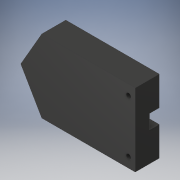
# Autodesk Inventor part: TARM05
Saved by Autodesk Inventor 2017 (Build 210142000, 142)
## iProperties
Created: 2018-10-19
Part Number: TARM05
Material: ABS Plastic
Document SubType Name: Modeling
Designer: Dell
Density: 1.06 g/cm^3
Appearance: Smooth - Black
Author: Dell
Autodesk Inventor part; units mm, degrees
ref_plane "YZ Plane" through (0, 0, 0) normal (1, 0, 0) x (0, 1, 0)
ref_plane "XZ Plane" through (0, 0, 0) normal (0, 1, 0) x (-1, 0, 0)
ref_plane "XY Plane" through (0, 0, 0) normal (0, 0, 1) x (1, 0, 0)
sketch "Sketch1" plane through (0, 0, 0) normal (0, 0, 1) x (1, 0, 0)
  line L0 (-56, 0) -> (-28, 48.4974)
  line L1 (-28, 48.4974) -> (28, 48.4974)
  line L2 (28, 48.4974) -> (56, 0)
  line L3 (56, 0) -> (28, -48.4974)
  line L4 (28, -48.4974) -> (-28, -48.4974)
  line L5 (-28, -48.4974) -> (-56, 0)
  line L6 (28, 48.4974) -> (76, 48.4974)
  line L7 (76, 48.4974) -> (76, -48.4974)
  line L8 (76, -48.4974) -> (28, -48.4974)
  point P0 (0, 0)
  point P1 (0, 0)
  dimension "d0" = 112
  dimension "d1" = 20
  constraints: 18 end point, 2 perpendicular, 1 coincident, 1 horizontal, 1 horizontal alignment, 13 other
  measures "d0" distance of L2.end L0.start
  measures "d1" distance from line of L2.end L7
extrude "Extrusion1" add sketch "Sketch1" along normal blind 5
sketch "Sketch2" plane through (0, 0, 0) normal (0, 0, -1) x (-1, 0, 0)
  line L0 (-76, 48.4974) -> (28, 48.4974) projected
  line L1 (28, 48.4974) -> (56, 0) projected
  line L2 (56, 0) -> (28, -48.4974) projected
  line L3 (28, -48.4974) -> (-76, -48.4974) projected
  line L4 (-76, 33.4974) -> (19.3397, 33.4974)
  line L5 (19.3397, 33.4974) -> (38.6795, 0)
  line L6 (38.6795, 0) -> (19.3397, -33.4974)
  line L7 (19.3397, -33.4974) -> (-76, -33.4974)
  line L8 (-76, -48.4974) -> (-76, 48.4974) projected
  line L9 (-76, -48.4974) -> (-76, 48.4974) projected
  line L10 (-76, 48.4974) -> (-56, 48.4974)
  line L11 (-56, 48.4974) -> (-56, -48.4974)
  line L12 (-56, -48.4974) -> (-76, -48.4974)
  line L13 (-76, -48.4974) -> (-76, 48.4974)
  line L14 (-76, 48.4974) -> (-76, 33.4974)
  line L15 (-76, -33.4974) -> (-76, -48.4974)
  point P0 (0, 0)
  dimension "d4" = 15
  dimension "d5" = 20
  constraints: 20 end point, 2 parallel, 1 collinear, 1 horizontal, 1 perpendicular, 1 point on line, 1 vertical, 3 other
  measures "d4" distance between parallel lines of L0 L4
  measures "d5" distance between parallel lines of L8 L11
extrude "Extrusion2" add sketch "Sketch2" along normal blind 15 contours L0 L11 L4 L8 | L0 L1 L2 L3 L11 L7 L6 L5 L4 | L4 L11 L7 L8 | L7 L11 L3 L8
sketch "Sketch3" plane through (0, 0, 5) normal (0, 0, 1) x (1, 0, 0)
  line L0 (76, 48.4974) -> (-28, 48.4974) projected
  line L1 (-28, 48.4974) -> (-56, 0) projected
  line L2 (-56, 0) -> (-28, -48.4974) projected
  line L3 (-28, -48.4974) -> (76, -48.4974) projected
  line L4 (76, -48.4974) -> (76, 48.4974) projected
  line L5 (66, -38.4974) -> (-22.2265, -38.4974)
  line L6 (-22.2265, -38.4974) -> (-44.453, 0)
  line L7 (-44.453, 0) -> (-22.2265, 38.4974)
  line L8 (-22.2265, 38.4974) -> (66, 38.4974)
  line L9 (66, 38.4974) -> (66, -38.4974)
  point P0 (0, 0)
  dimension "d8" = 10
  constraints: 10 end point, 4 other
  measures "d8" distance between parallel lines of L3 L5
extrude "Extrusion3" cut sketch "Sketch3" against normal through all
sketch "Sketch4" plane through (0, 0, 0) normal (0, 0, -1) x (-1, 0, 0)
  line L0 (-66, -38.4974) -> (-76, -38.4974)
  line L1 (-76, -38.4974) -> (-76, 38.4974)
  line L2 (-76, 38.4974) -> (-66, 38.4974)
  line L3 (-66, 38.4974) -> (-66, -38.4974)
  point P0 (0, 0)
  dimension "d11" = 10
  constraints: 8 end point, 2 parallel, 1 coincident, 1 horizontal, 1 perpendicular
  measures "d11" distance of L0.start L0.end
extrude "Extrusion4" add sketch "Sketch4" along normal blind 15 and the other way blind 5
sketch "Sketch5" plane through (0, 0, 0) normal (0, 0, -1) x (-1, 0, 0)
  line L0 (-56, 33.4974) -> (-56, -33.4974) projected
  line L1 (-56, -33.4974) -> (19.3397, -33.4974) projected
  line L2 (19.3397, -33.4974) -> (38.6795, 0) projected
  line L3 (38.6795, 0) -> (19.3397, 33.4974) projected
  line L4 (19.3397, 33.4974) -> (-56, 33.4974) projected
  point P0 (0, 0)
extrude "Extrusion5" add sketch "Sketch5" along normal blind 5
sketch "Sketch7" plane through (0, 0, 5) normal (0, 0, 1) x (1, 0, 0)
  line L0 (76, 38.4974) -> (-22.2265, 38.4974) projected
  line L1 (-22.2265, 38.4974) -> (-44.453, 0) projected
  line L2 (-44.453, 0) -> (-22.2265, -38.4974) projected
  line L3 (-22.2265, -38.4974) -> (76, -38.4974) projected
  line L4 (76, -38.4974) -> (76, 38.4974) projected
  point P0 (0, 0)
extrude "Extrusion6" cut sketch "Sketch7" against normal blind 5
sketch "Sketch8" plane through (56, -33.4974, -15) normal (-1, 0, 0) x (0, 0, 1)
  line L0 (10, 0) -> (10, 66.9948) projected
  line L1 (0, 66.9948) -> (10, 66.9948) projected
  line L2 (0, 0) -> (0, 66.9948) projected
  line L3 (10, 0) -> (0, 0) projected
  line L4 (0, 71.9948) -> (0, -5) projected
  line L5 (0, 25.9974) -> (10, 25.9974)
  line L6 (10, 25.9974) -> (10, 40.9974)
  line L7 (10, 40.9974) -> (0, 40.9974)
  line L8 (0, 40.9974) -> (0, 25.9974)
  point P0 (15, 33.4974)
  point P1 (10, 33.4974)
  dimension "d20" = 15
  constraints: 8 end point, 2 parallel, 2 point on line, 1 horizontal, 1 horizontal alignment, 1 midpoint, 1 perpendicular
  measures "d20" distance between parallel lines of L7 L5
extrude "Extrusion7" cut sketch "Sketch8" against normal through all contours L5 L2 L7 L0
sketch "Sketch9" plane through (0, 0, -15) normal (0, 0, -1) x (-1, 0, 0)
  line L0 (-76, -7.5) -> (-76, 7.5) construction
  line L1 (-56, -7.5) -> (-76, -7.5) construction
  line L2 (-68.5, -27.5) -> (-68.5, 27.5) construction
  circle A0 centre (-68.5, -27.5) radius 2.5
  circle A1 centre (-68.5, 27.5) radius 2.5
  point P0 (0, 0)
  point P1 (-68.5, 0)
  point P2 (-76, 0)
  dimension "d23" = 55
  dimension "d24" = 5
  dimension "d25" = 5
  dimension "d32" = 7.5
  constraints: 2 centre point, 2 coincident, 2 end point, 2 midpoint, 1 horizontal alignment, 1 vertical
  measures "d23" distance of L2.start L2.end
  measures "d24" diameter of A0
  measures "d25" diameter of A1
  measures "d32" distance between parallel lines of L2 L0
extrude "Extrusion8" cut sketch "Sketch9" against normal through all
sketch "Sketch10" plane through (0, 0, 0) normal (0, 0, 1) x (1, 0, 0)
  circle A0 centre (68.5, -27.5) radius 2.5 projected
  circle A1 centre (68.5, 27.5) radius 2.5 projected
  line L0 (-22.2265, 38.4974) -> (76, 38.4974) projected
  line L1 (-44.453, 0) -> (-22.2265, 38.4974) projected
  line L2 (-22.2265, -38.4974) -> (-44.453, 0) projected
  line L3 (76, -38.4974) -> (-22.2265, -38.4974) projected
  line L4 (76, 38.4974) -> (76, -38.4974) projected
  line L5 (-43.8756, 0) -> (-21.9378, 37.9974)
  line L6 (-21.9378, 37.9974) -> (75.5, 37.9974)
  line L7 (75.5, 37.9974) -> (75.5, -37.9974)
  line L8 (75.5, -37.9974) -> (-21.9378, -37.9974)
  line L9 (-21.9378, -37.9974) -> (-43.8756, 0)
  point P0 (0, 0)
  dimension "d29" = 0.5
  constraints: 10 end point, 4 other
  measures "d29" distance between parallel lines of L2 L9
extrude "Extrusion9" cut sketch "Sketch10" against normal through all contours L0 L4 L3 L2 L1
sketch "Sketch12" plane through (0, 0, -15) normal (0, 0, -1) x (-1, 0, 0)
  line L0 (-75.5, 37.9974) -> (-75.5, 7.5) projected
  line L1 (-75.5, 7.5) -> (-56, 7.5) projected
  line L2 (-56, 7.5) -> (-56, 33.4974) projected
  line L3 (-56, 33.4974) -> (19.3397, 33.4974) projected
  line L4 (19.3397, 33.4974) -> (38.6795, 0) projected
  line L5 (38.6795, 0) -> (19.3397, -33.4974) projected
  line L6 (19.3397, -33.4974) -> (-56, -33.4974) projected
  line L7 (-56, -33.4974) -> (-56, -7.5) projected
  line L8 (-56, -7.5) -> (-75.5, -7.5) projected
  line L9 (-75.5, -7.5) -> (-75.5, -37.9974) projected
  line L10 (-75.5, -37.9974) -> (21.9378, -37.9974) projected
  line L11 (21.9378, -37.9974) -> (43.8756, 0) projected
  line L12 (43.8756, 0) -> (21.9378, 37.9974) projected
  line L13 (21.9378, 37.9974) -> (-75.5, 37.9974) projected
  circle A0 centre (-68.5, -27.5) radius 2.5 projected
  circle A1 centre (-68.5, 27.5) radius 2.5 projected
  point P0 (0, 0)
extrude "Extrusion11" add sketch "Sketch12" along normal blind 10
sketch "Sketch13" plane through (75.5, -37.9974, 0) normal (1, 0, 0) x (0, 0, -1)
  line L0 (5, 45.4974) -> (5, 30.4974) projected
  line L1 (25, 45.4974) -> (5, 45.4974) projected
  line L2 (5, 45.4974) -> (15, 45.4974)
  line L3 (15, 45.4974) -> (15, 30.4974)
  line L4 (15, 30.4974) -> (5, 30.4974)
  line L5 (5, 30.4974) -> (5, 45.4974)
  line L6 (5, 30.4974) -> (25, 30.4974) projected
  point P0 (0, 37.9974)
  dimension "d39" = 10
  constraints: 8 end point, 2 parallel, 1 horizontal, 1 midpoint, 1 perpendicular
  measures "d39" distance between parallel lines of L0 L3
extrude "Extrusion12" add sketch "Sketch13" against normal blind 19.5
body "Solid1"
